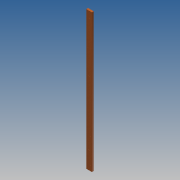
# Autodesk Inventor part: 2p2psv
Saved by Autodesk Inventor 2014 SP1 (Build 180222100, 222)
## iProperties
Created: 2013-09-03
Part Number: 2p2psv
Material: Wood (Cherry)
Document SubType Name: Modeling
Designer: David DeBoer
Mass: 3352.84 g
Surface Area: 5127.86 cm^2
Volume: 6705.68 cm^3
Density: 0.5 g/cm^3
Description: Pole stand vertical support
Appearance: Cherry - Natural Low Gloss
Author: Dave
Autodesk Inventor part; units mm, degrees
ref_plane "YZ Plane" through (0, 0, 0) normal (1, 0, 0) x (0, 1, 0)
ref_plane "XZ Plane" through (0, 0, 0) normal (0, 1, 0) x (-1, 0, 0)
ref_plane "XY Plane" through (0, 0, 0) normal (0, 0, 1) x (1, 0, 0)
sketch "Sketch1" plane through (0, 0, 0) normal (0, 1, 0) x (-1, 0, 0)
  line L0 (0, 0) -> (114, 0)
  line L1 (114, 0) -> (114, 38)
  line L2 (114, 38) -> (0, 38)
  line L3 (0, 38) -> (0, 0)
  dimension "d0" = 114
  dimension "d1" = 38
  constraints: 8 end point, 2 parallel, 1 horizontal, 1 perpendicular
  measures "d0" distance of L0.start L0.end
  measures "d1" distance of L2.end L0.start
extrude "Extrusion1" add sketch "Sketch1" along normal blind 2794
sketch "Sketch3" plane through (-114, 0, 38) normal (0, 0, 1) x (1, 0, 0)
  line L0 (0, 0) -> (114, 0) projected
  line L1 (0, 0) -> (0, 2794) projected
  circle A0 centre (28.5, 101.6) radius 5.7238
  circle A1 centre (85.5, 101.6) radius 5.7238
  circle A2 centre (28.5, 609.6) radius 5.7238
  circle A3 centre (85.5, 609.6) radius 5.7238
  dimension "d28" = 101.6
  dimension "d29" = 28.5
  dimension "d32" = 57
  dimension "d35" = 508
  constraints: 4 centre point, 1 horizontal, 1 vertical, 6 other
  measures "d28" distance from line of L0 A0.centre
  measures "d29" distance from line of A0.centre L1
  measures "d32" distance of A0.centre A1.centre
  measures "d35" distance of A0.centre A2.centre
hole "rimArm" at (-85.5, 609.6, 38) at (-28.5, 609.6, 38) at (-85.5, 101.6, 38) at (-28.5, 101.6, 38) direction (0, 0, -1) diameter 6.35 end through all
sketch "Sketch4" plane through (-114, 0, 38) normal (0, 0, 1) x (1, 0, 0)
  line L0 (0, 2794) -> (114, 2794) projected
  line L1 (0, 0) -> (0, 2794) projected
  circle A0 centre (28.5, 2774.95) radius 4.8454
  circle A1 centre (85.5, 2774.95) radius 4.8454
  circle A2 centre (28.5, 2139.95) radius 4.8454
  circle A3 centre (85.5, 2139.95) radius 4.8454
  dimension "d45" = 19.05
  dimension "d48" = 57
  dimension "d51" = 635
  dimension "d71" = 28.5
  constraints: 4 centre point, 1 horizontal, 1 vertical, 6 other
  measures "d45" distance from line of A0.centre L0
  measures "d48" distance of A0.centre A1.centre
  measures "d51" distance of A0.centre A2.centre
  measures "d71" distance from line of A0.centre L1
hole "screenArm" at (-85.5, 2774.95, 38) at (-28.5, 2774.95, 38) at (-28.5, 2139.95, 38) at (-85.5, 2139.95, 38) direction (0, 0, -1) diameter 6.7564 end through all clearance for "Flat Head Machine Screw (82)" size "1/4" standard "Ansi Unified Screw Threads"
sketch "Sketch5" plane through (-114, 0, 38) normal (0, 0, 1) x (1, 0, 0)
  line L0 (0, 0) -> (114, 0) projected
  line L1 (0, 2794) -> (114, 2794) projected
  circle A0 centre (57, 2667) radius 8.4367
  circle A1 centre (57, 1651) radius 12.5456
  circle A2 centre (57, 355.6) radius 11.5895
  line L2 (0, 0) -> (0, 2794) projected
  dimension "d61" = 127
  dimension "d62" = 355.6
  dimension "d70" = 1651
  dimension "d72" = 57
  dimension "d73" = 57
  dimension "d74" = 57
  constraints: 3 centre point
  measures "d61" distance from line of L1 A0.centre
  measures "d62" distance from line of L0 A2.centre
  measures "d70" distance from line of L0 A1.centre
  measures "d72" distance from line of A0.centre L2
  measures "d73" distance from line of A1.centre L2
  measures "d74" distance from line of A2.centre L2
hole "poleAttach" at (-57, 2667, 38) at (-57, 1651, 38) at (-57, 355.6, 38) direction (0, 0, -1) diameter 10.0838 end through all clearance for "Flat Head Machine Screw (82)" size "3/8" standard "Ansi Unified Screw Threads"
equation "\"d29\" = 0.25 * d0"
equation "\"d32\" = 0.5 * d0"
equation "\"d48\" = 0.5 * d0"
equation "\"d71\" = 0.25 * d0"
equation "\"d72\" = 0.5 * d0"
equation "\"d73\" = 0.5 * d0"
equation "\"d74\" = 0.5 * d0"
body "Solid1"
